Autodesk Fusion 360 part; units mm, degrees
(part 2 of 6)
  spline S17 degree 5 poles (13.6147, 25.8496) (13.6143, 25.8607) (13.6137, 25.8829) (13.6125, 25.9162) (13.6109, 25.9605) (13.6086, 26.0158) (13.6061, 26.0711) (13.6034, 26.1262) (13.6004, 26.1813) (13.5971, 26.2363) (13.5936, 26.2912) (13.5899, 26.346) (13.586, 26.4008) (13.5817, 26.4554) (13.5773, 26.51) (13.5726, 26.5644) (13.5676, 26.6188) (13.5624, 26.6731) (13.5569, 26.7273) (13.5512, 26.7813) (13.5453, 26.8353) (13.539, 26.8892) (13.5325, 26.943) (13.5258, 26.9966) (13.5188, 27.0502) (13.5115, 27.1037) (13.504, 27.157) (13.4962, 27.2102) (13.4882, 27.2634) (13.4798, 27.3164) (13.4712, 27.3693) (13.4623, 27.422) (13.4532, 27.4747) (13.4438, 27.5272) (13.4341, 27.5796) (13.4241, 27.6319) (13.4138, 27.684) (13.4032, 27.736) (13.3924, 27.7879) (13.3812, 27.8397) (13.3698, 27.8913) (13.3581, 27.9427) (13.346, 27.994) (13.3337, 28.0452) (13.321, 28.0962) (13.308, 28.147) (13.2947, 28.1977) (13.2811, 28.2483) (13.2672, 28.2986) (13.253, 28.3488) (13.2384, 28.3989) (13.2234, 28.4487) (13.2081, 28.4983) (13.1924, 28.5478) (13.1763, 28.597) (13.1599, 28.646) (13.1431, 28.6949) (13.126, 28.7436) (13.1086, 28.7921) (13.0908, 28.8403) (13.0724, 28.8883) (13.0536, 28.936) (13.0341, 28.9833) (13.014, 29.0303) (12.9935, 29.0769) (12.9725, 29.1234) (12.9513, 29.1696) (12.9298, 29.2157) (12.9079, 29.2615) (12.8852, 29.3069) (12.8613, 29.3515) (12.8409, 29.3863) (12.8246, 29.4119) (12.8134, 29.4287) (12.8076, 29.437) knots -1 -1 -1 -1 -1 -1 -0.98571429 -0.97142857 -0.95714286 -0.94285714 -0.92857143 -0.91428571 -0.9 -0.88571429 -0.87142857 -0.85714286 -0.84285714 -0.82857143 -0.81428571 -0.8 -0.78571429 -0.77142857 -0.75714286 -0.74285714 -0.72857143 -0.71428571 -0.7 -0.68571429 -0.67142857 -0.65714286 -0.64285714 -0.62857143 -0.61428571 -0.6 -0.58571429 -0.57142857 -0.55714286 -0.54285714 -0.52857143 -0.51428571 -0.5 -0.48571429 -0.47142857 -0.45714286 -0.44285714 -0.42857143 -0.41428571 -0.4 -0.38571429 -0.37142857 -0.35714286 -0.34285714 -0.32857143 -0.31428571 -0.3 -0.28571429 -0.27142857 -0.25714286 -0.24285714 -0.22857143 -0.21428571 -0.2 -0.18571429 -0.17142857 -0.15714286 -0.14285714 -0.12857143 -0.11428571 -0.1 -0.08571429 -0.07142857 -0.05714286 -0.04285714 -0.02857143 -0.01428571 0 0 0 0 0 0
  line L17 (12.8076, 29.437) -> (12.7927, 29.4587)
  arc A35 (13.0124, 30.8231) -> (12.7927, 29.4587) centre (13.6162, 30.026) ccw
  arc A36 (13.0124, 30.8231) -> (13.2238, 30.9853) centre (0, 48) ccw
  arc A37 (14.5985, 30.8444) -> (13.2238, 30.9853) centre (13.8374, 30.1957) ccw
  line L18 (14.5985, 30.8444) -> (14.6156, 30.8243)
  spline S18 degree 5 poles (14.6156, 30.8243) (14.6222, 30.8166) (14.6355, 30.8014) (14.656, 30.7791) (14.6843, 30.7503) (14.7212, 30.7157) (14.7592, 30.6821) (14.7977, 30.6491) (14.8367, 30.6164) (14.8759, 30.5839) (14.9153, 30.5516) (14.9551, 30.5197) (14.9953, 30.4881) (15.0359, 30.4571) (15.0771, 30.4265) (15.1187, 30.3964) (15.1607, 30.3667) (15.203, 30.3373) (15.2456, 30.3082) (15.2885, 30.2794) (15.3316, 30.2508) (15.375, 30.2225) (15.4187, 30.1946) (15.4626, 30.1669) (15.5069, 30.1396) (15.5514, 30.1125) (15.5963, 30.0858) (15.6413, 30.0593) (15.6866, 30.0331) (15.7321, 30.0071) (15.7779, 29.9814) (15.8239, 29.956) (15.8701, 29.9308) (15.9165, 29.9059) (15.9632, 29.8812) (16.0101, 29.8568) (16.0572, 29.8327) (16.1045, 29.8088) (16.152, 29.7851) (16.1997, 29.7617) (16.2476, 29.7385) (16.2957, 29.7156) (16.344, 29.6929) (16.3925, 29.6704) (16.4412, 29.6482) (16.49, 29.6262) (16.5391, 29.6044) (16.5883, 29.5829) (16.6377, 29.5616) (16.6873, 29.5405) (16.737, 29.5196) (16.787, 29.499) (16.8371, 29.4786) (16.8873, 29.4584) (16.9377, 29.4385) (16.9883, 29.4187) (17.0391, 29.3992) (17.09, 29.3799) (17.1411, 29.3608) (17.1923, 29.342) (17.2437, 29.3233) (17.2953, 29.3049) (17.3469, 29.2867) (17.3988, 29.2687) (17.4508, 29.2509) (17.5029, 29.2333) (17.5552, 29.216) (17.6076, 29.1988) (17.6602, 29.1819) (17.7129, 29.1652) (17.7658, 29.1486) (17.8081, 29.1356) (17.84, 29.1259) (17.8613, 29.1195) (17.8719, 29.1163) knots 0 0 0 0 0 0 0.01428571 0.02857143 0.04285714 0.05714286 0.07142857 0.08571429 0.1 0.11428571 0.12857143 0.14285714 0.15714286 0.17142857 0.18571429 0.2 0.21428571 0.22857143 0.24285714 0.25714286 0.27142857 0.28571429 0.3 0.31428571 0.32857143 0.34285714 0.35714286 0.37142857 0.38571429 0.4 0.41428571 0.42857143 0.44285714 0.45714286 0.47142857 0.48571429 0.5 0.51428571 0.52857143 0.54285714 0.55714286 0.57142857 0.58571429 0.6 0.61428571 0.62857143 0.64285714 0.65714286 0.67142857 0.68571429 0.7 0.71428571 0.72857143 0.74285714 0.75714286 0.77142857 0.78571429 0.8 0.81428571 0.82857143 0.84285714 0.85714286 0.87142857 0.88571429 0.9 0.91428571 0.92857143 0.94285714 0.95714286 0.97142857 0.98571429 1 1 1 1 1 1
  arc A38 (17.8719, 29.1163) -> (18.8837, 30.1281) centre (0, 48) ccw
  spline S19 degree 5 poles (18.8837, 30.1281) (18.8805, 30.1387) (18.8741, 30.16) (18.8644, 30.1919) (18.8514, 30.2342) (18.8348, 30.2871) (18.8181, 30.3398) (18.8012, 30.3924) (18.784, 30.4448) (18.7667, 30.4971) (18.7491, 30.5492) (18.7313, 30.6012) (18.7133, 30.6531) (18.6951, 30.7047) (18.6767, 30.7563) (18.658, 30.8077) (18.6392, 30.8589) (18.6201, 30.91) (18.6008, 30.9609) (18.5813, 31.0117) (18.5615, 31.0623) (18.5416, 31.1127) (18.5214, 31.1629) (18.501, 31.213) (18.4804, 31.263) (18.4595, 31.3127) (18.4384, 31.3623) (18.4171, 31.4117) (18.3956, 31.4609) (18.3738, 31.51) (18.3518, 31.5588) (18.3296, 31.6075) (18.3071, 31.656) (18.2844, 31.7043) (18.2615, 31.7524) (18.2383, 31.8003) (18.2149, 31.848) (18.1912, 31.8955) (18.1673, 31.9428) (18.1432, 31.9899) (18.1188, 32.0368) (18.0941, 32.0835) (18.0692, 32.1299) (18.044, 32.1761) (18.0186, 32.2221) (17.9929, 32.2679) (17.9669, 32.3134) (17.9407, 32.3587) (17.9142, 32.4037) (17.8875, 32.4486) (17.8604, 32.4931) (17.8331, 32.5374) (17.8054, 32.5813) (17.7775, 32.625) (17.7492, 32.6684) (17.7206, 32.7115) (17.6918, 32.7544) (17.6627, 32.797) (17.6333, 32.8393) (17.6036, 32.8813) (17.5735, 32.9229) (17.5429, 32.9641) (17.5119, 33.0047) (17.4803, 33.0449) (17.4484, 33.0847) (17.4161, 33.1241) (17.3836, 33.1633) (17.3509, 33.2023) (17.3179, 33.2408) (17.2843, 33.2788) (17.2497, 33.3157) (17.2209, 33.344) (17.1986, 33.3645) (17.1834, 33.3778) (17.1757, 33.3844) knots -1 -1 -1 -1 -1 -1 -0.98571429 -0.97142857 -0.95714286 -0.94285714 -0.92857143 -0.91428571 -0.9 -0.88571429 -0.87142857 -0.85714286 -0.84285714 -0.82857143 -0.81428571 -0.8 -0.78571429 -0.77142857 -0.75714286 -0.74285714 -0.72857143 -0.71428571 -0.7 -0.68571429 -0.67142857 -0.65714286 -0.64285714 -0.62857143 -0.61428571 -0.6 -0.58571429 -0.57142857 -0.55714286 -0.54285714 -0.52857143 -0.51428571 -0.5 -0.48571429 -0.47142857 -0.45714286 -0.44285714 -0.42857143 -0.41428571 -0.4 -0.38571429 -0.37142857 -0.35714286 -0.34285714 -0.32857143 -0.31428571 -0.3 -0.28571429 -0.27142857 -0.25714286 -0.24285714 -0.22857143 -0.21428571 -0.2 -0.18571429 -0.17142857 -0.15714286 -0.14285714 -0.12857143 -0.11428571 -0.1 -0.08571429 -0.07142857 -0.05714286 -0.04285714 -0.02857143 -0.01428571 0 0 0 0 0 0
  line L19 (17.1757, 33.3844) -> (17.1556, 33.4015)
  arc A39 (17.0147, 34.7762) -> (17.1556, 33.4015) centre (17.8043, 34.1626) ccw
  arc A40 (17.0147, 34.7762) -> (17.1769, 34.9876) centre (0, 48) ccw
  arc A41 (18.5413, 35.2073) -> (17.1769, 34.9876) centre (17.974, 34.3838) ccw
  line L20 (18.5413, 35.2073) -> (18.563, 35.1924)
  spline S20 degree 5 poles (18.563, 35.1924) (18.5713, 35.1866) (18.5881, 35.1754) (18.6137, 35.1591) (18.6485, 35.1387) (18.6931, 35.1148) (18.7385, 35.0921) (18.7843, 35.0702) (18.8304, 35.0487) (18.8766, 35.0275) (18.9231, 35.0065) (18.9697, 34.986) (19.0167, 34.9659) (19.064, 34.9464) (19.1117, 34.9276) (19.1597, 34.9092) (19.2079, 34.8914) (19.2564, 34.874) (19.3051, 34.8569) (19.354, 34.8401) (19.403, 34.8237) (19.4522, 34.8076) (19.5017, 34.7919) (19.5513, 34.7766) (19.6011, 34.7616) (19.6512, 34.747) (19.7014, 34.7328) (19.7517, 34.7189) (19.8023, 34.7053) (19.853, 34.692) (19.9038, 34.679) (19.9548, 34.6663) (20.006, 34.654) (20.0573, 34.6419) (20.1087, 34.6302) (20.1603, 34.6188) (20.2121, 34.6076) (20.264, 34.5968) (20.316, 34.5862) (20.3681, 34.5759) (20.4204, 34.5659) (20.4728, 34.5562) (20.5253, 34.5468) (20.578, 34.5377) (20.6307, 34.5288) (20.6836, 34.5202) (20.7366, 34.5118) (20.7898, 34.5038) (20.843, 34.496) (20.8963, 34.4885) (20.9498, 34.4812) (21.0034, 34.4742) (21.057, 34.4675) (21.1108, 34.461) (21.1647, 34.4547) (21.2187, 34.4488) (21.2727, 34.4431) (21.3269, 34.4376) (21.3812, 34.4324) (21.4356, 34.4274) (21.49, 34.4227) (21.5446, 34.4183) (21.5992, 34.414) (21.654, 34.4101) (21.7088, 34.4064) (21.7637, 34.4029) (21.8187, 34.3996) (21.8738, 34.3966) (21.9289, 34.3939) (21.9842, 34.3914) (22.0395, 34.3891) (22.0838, 34.3875) (22.1171, 34.3863) (22.1393, 34.3857) (22.1504, 34.3853) knots 0 0 0 0 0 0 0.01428571 0.02857143 0.04285714 0.05714286 0.07142857 0.08571429 0.1 0.11428571 0.12857143 0.14285714 0.15714286 0.17142857 0.18571429 0.2 0.21428571 0.22857143 0.24285714 0.25714286 0.27142857 0.28571429 0.3 0.31428571 0.32857143 0.34285714 0.35714286 0.37142857 0.38571429 0.4 0.41428571 0.42857143 0.44285714 0.45714286 0.47142857 0.48571429 0.5 0.51428571 0.52857143 0.54285714 0.55714286 0.57142857 0.58571429 0.6 0.61428571 0.62857143 0.64285714 0.65714286 0.67142857 0.68571429 0.7 0.71428571 0.72857143 0.74285714 0.75714286 0.77142857 0.78571429 0.8 0.81428571 0.82857143 0.84285714 0.85714286 0.87142857 0.88571429 0.9 0.91428571 0.92857143 0.94285714 0.95714286 0.97142857 0.98571429 1 1 1 1 1 1
  arc A42 (22.1504, 34.3853) -> (22.8659, 35.6245) centre (0, 48) ccw
  spline S21 degree 5 poles (22.8659, 35.6245) (22.86, 35.634) (22.8483, 35.6529) (22.8307, 35.6811) (22.8071, 35.7187) (22.7775, 35.7655) (22.7477, 35.812) (22.7177, 35.8584) (22.6876, 35.9046) (22.6573, 35.9507) (22.6268, 35.9965) (22.5962, 36.0421) (22.5654, 36.0875) (22.5344, 36.1327) (22.5033, 36.1777) (22.472, 36.2225) (22.4405, 36.2671) (22.4088, 36.3115) (22.377, 36.3557) (22.345, 36.3997) (22.3129, 36.4435) (22.2805, 36.487) (22.248, 36.5303) (22.2154, 36.5735) (22.1825, 36.6163) (22.1495, 36.659) (22.1163, 36.7014) (22.0829, 36.7436) (22.0494, 36.7856) (22.0157, 36.8274) (21.9818, 36.8689) (21.9477, 36.9101) (21.9135, 36.9512) (21.879, 36.9919) (21.8444, 37.0325) (21.8096, 37.0727) (21.7747, 37.1127) (21.7395, 37.1525) (21.7042, 37.192) (21.6687, 37.2313) (21.633, 37.2702) (21.5971, 37.3089) (21.561, 37.3473) (21.5247, 37.3854) (21.4882, 37.4233) (21.4516, 37.4608) (21.4147, 37.4981) (21.3777, 37.5351) (21.3404, 37.5717) (21.303, 37.6081) (21.2653, 37.6441) (21.2275, 37.6798) (21.1894, 37.7151) (21.1511, 37.7501) (21.1125, 37.7847) (21.0738, 37.8189) (21.0348, 37.8529) (20.9957, 37.8865) (20.9563, 37.9197) (20.9168, 37.9526) (20.8769, 37.985) (20.8367, 38.0168) (20.7962, 38.0481) (20.7554, 38.0787) (20.7142, 38.1089) (20.6728, 38.1386) (20.6313, 38.1681) (20.5897, 38.1972) (20.5478, 38.2259) (20.5055, 38.2539) (20.4625, 38.2806) (20.4274, 38.3005) (20.4005, 38.3145) (20.3824, 38.3235) (20.3732, 38.3278) knots -1 -1 -1 -1 -1 -1 -0.98571429 -0.97142857 -0.95714286 -0.94285714 -0.92857143 -0.91428571 -0.9 -0.88571429 -0.87142857 -0.85714286 -0.84285714 -0.82857143 -0.81428571 -0.8 -0.78571429 -0.77142857 -0.75714286 -0.74285714 -0.72857143 -0.71428571 -0.7 -0.68571429 -0.67142857 -0.65714286 -0.64285714 -0.62857143 -0.61428571 -0.6 -0.58571429 -0.57142857 -0.55714286 -0.54285714 -0.52857143 -0.51428571 -0.5 -0.48571429 -0.47142857 -0.45714286 -0.44285714 -0.42857143 -0.41428571 -0.4 -0.38571429 -0.37142857 -0.35714286 -0.34285714 -0.32857143 -0.31428571 -0.3 -0.28571429 -0.27142857 -0.25714286 -0.24285714 -0.22857143 -0.21428571 -0.2 -0.18571429 -0.17142857 -0.15714286 -0.14285714 -0.12857143 -0.11428571 -0.1 -0.08571429 -0.07142857 -0.05714286 -0.04285714 -0.02857143 -0.01428571 0 0 0 0 0 0
  line L21 (20.3732, 38.3278) -> (20.3494, 38.3391)
  arc A43 (19.8575, 39.6305) -> (20.3494, 38.3391) centre (20.779, 39.2422) ccw
  arc A44 (19.8575, 39.6305) -> (19.9595, 39.8767) centre (0, 48) ccw
  arc A45 (21.2205, 40.4421) -> (19.9595, 39.8767) centre (20.8857, 39.4998) ccw
  line L22 (21.2205, 40.4421) -> (21.2453, 40.4332)
  spline S22 degree 5 poles (21.2453, 40.4332) (21.2549, 40.4298) (21.274, 40.4233) (21.3029, 40.4142) (21.3419, 40.4035) (21.3911, 40.392) (21.4408, 40.3818) (21.4907, 40.3725) (21.5408, 40.3637) (21.591, 40.3551) (21.6412, 40.3469) (21.6916, 40.3391) (21.7422, 40.3319) (21.7929, 40.3254) (21.8439, 40.3195) (21.895, 40.3142) (21.9462, 40.3094) (21.9975, 40.3052) (22.049, 40.3012) (22.1005, 40.2977) (22.1521, 40.2945) (22.2039, 40.2917) (22.2557, 40.2894) (22.3076, 40.2874) (22.3596, 40.2859) (22.4117, 40.2847) (22.4639, 40.2839) (22.5161, 40.2835) (22.5685, 40.2835) (22.6209, 40.2838) (22.6733, 40.2844) (22.7259, 40.2854) (22.7785, 40.2867) (22.8312, 40.2883) (22.8839, 40.2903) (22.9367, 40.2926) (22.9896, 40.2952) (23.0425, 40.2982) (23.0955, 40.3014) (23.1485, 40.305) (23.2016, 40.3089) (23.2547, 40.3131) (23.3079, 40.3176) (23.3611, 40.3223) (23.4144, 40.3274) (23.4677, 40.3328) (23.521, 40.3385) (23.5744, 40.3444) (23.6279, 40.3507) (23.6814, 40.3572) (23.7349, 40.364) (23.7884, 40.3711) (23.842, 40.3785) (23.8956, 40.3862) (23.9493, 40.3941) (24.003, 40.4023) (24.0567, 40.4108) (24.1104, 40.4195) (24.1642, 40.4286) (24.218, 40.4378) (24.2718, 40.4474) (24.3257, 40.4572) (24.3796, 40.4673) (24.4335, 40.4776) (24.4874, 40.4882) (24.5413, 40.499) (24.5953, 40.5101) (24.6492, 40.5215) (24.7032, 40.5331) (24.7573, 40.545) (24.8113, 40.5571) (24.8545, 40.567) (24.8869, 40.5745) (24.9086, 40.5796) (24.9194, 40.5822) knots 0 0 0 0 0 0 0.01428571 0.02857143 0.04285714 0.05714286 0.07142857 0.08571429 0.1 0.11428571 0.12857143 0.14285714 0.15714286 0.17142857 0.18571429 0.2 0.21428571 0.22857143 0.24285714 0.25714286 0.27142857 0.28571429 0.3 0.31428571 0.32857143 0.34285714 0.35714286 0.37142857 0.38571429 0.4 0.41428571 0.42857143 0.44285714 0.45714286 0.47142857 0.48571429 0.5 0.51428571 0.52857143 0.54285714 0.55714286 0.57142857 0.58571429 0.6 0.61428571 0.62857143 0.64285714 0.65714286 0.67142857 0.68571429 0.7 0.71428571 0.72857143 0.74285714 0.75714286 0.77142857 0.78571429 0.8 0.81428571 0.82857143 0.84285714 0.85714286 0.87142857 0.88571429 0.9 0.91428571 0.92857143 0.94285714 0.95714286 0.97142857 0.98571429 1 1 1 1 1 1
  arc A46 (24.9194, 40.5822) -> (25.2897, 41.9643) centre (0, 48) ccw
  spline S23 degree 5 poles (25.2897, 41.9643) (25.2816, 41.9719) (25.2655, 41.9872) (25.2411, 42.0099) (25.2086, 42.0401) (25.1679, 42.0776) (25.1271, 42.1149) (25.0861, 42.1519) (25.0451, 42.1888) (25.0039, 42.2254) (24.9626, 42.2617) (24.9212, 42.2979) (24.8797, 42.3338) (24.8381, 42.3694) (24.7963, 42.4048) (24.7545, 42.44) (24.7125, 42.475) (24.6705, 42.5097) (24.6283, 42.5441) (24.586, 42.5783) (24.5436, 42.6122) (24.5011, 42.6459) (24.4585, 42.6794) (24.4158, 42.7126) (24.373, 42.7455) (24.33, 42.7782) (24.287, 42.8105) (24.2438, 42.8427) (24.2006, 42.8745) (24.1572, 42.9061) (24.1137, 42.9375) (24.0701, 42.9685) (24.0264, 42.9993) (23.9826, 43.0297) (23.9387, 43.0599) (23.8947, 43.0898) (23.8505, 43.1194) (23.8063, 43.1487) (23.7619, 43.1777) (23.7175, 43.2065) (23.6729, 43.2349) (23.6282, 43.2629) (23.5834, 43.2907) (23.5385, 43.3181) (23.4935, 43.3452) (23.4484, 43.372) (23.4031, 43.3985) (23.3578, 43.4246) (23.3123, 43.4504) (23.2667, 43.4758) (23.221, 43.5008) (23.1752, 43.5255) (23.1293, 43.5498) (23.0832, 43.5736) (23.037, 43.5971) (22.9908, 43.6201) (22.9444, 43.6428) (22.8979, 43.6652) (22.8512, 43.6871) (22.8045, 43.7086) (22.7576, 43.7296) (22.7106, 43.75) (22.6633, 43.7696) (22.6159, 43.7887) (22.5684, 43.8071) (22.5207, 43.8252) (22.473, 43.8429) (22.4252, 43.8602) (22.3773, 43.8771) (22.3292, 43.8932) (22.2808, 43.9078) (22.2417, 43.918) (22.2122, 43.9246) (22.1923, 43.9285) (22.1824, 43.9304) knots -1 -1 -1 -1 -1 -1 -0.98571429 -0.97142857 -0.95714286 -0.94285714 -0.92857143 -0.91428571 -0.9 -0.88571429 -0.87142857 -0.85714286 -0.84285714 -0.82857143 -0.81428571 -0.8 -0.78571429 -0.77142857 -0.75714286 -0.74285714 -0.72857143 -0.71428571 -0.7 -0.68571429 -0.67142857 -0.65714286 -0.64285714 -0.62857143 -0.61428571 -0.6 -0.58571429 -0.57142857 -0.55714286 -0.54285714 -0.52857143 -0.51428571 -0.5 -0.48571429 -0.47142857 -0.45714286 -0.44285714 -0.42857143 -0.41428571 -0.4 -0.38571429 -0.37142857 -0.35714286 -0.34285714 -0.32857143 -0.31428571 -0.3 -0.28571429 -0.27142857 -0.25714286 -0.24285714 -0.22857143 -0.21428571 -0.2 -0.18571429 -0.17142857 -0.15714286 -0.14285714 -0.12857143 -0.11428571 -0.1 -0.08571429 -0.07142857 -0.05714286 -0.04285714 -0.02857143 -0.01428571 0 0 0 0 0 0
  line L23 (22.1824, 43.9304) -> (22.1564, 43.9351)
  arc A47 (21.347, 45.0552) -> (22.1564, 43.9351) centre (22.3377, 44.9186) ccw
  arc A48 (21.347, 45.0552) -> (21.3818, 45.3194) centre (0, 48) ccw
  arc A49 (22.4535, 46.1918) -> (21.3818, 45.3194) centre (22.3741, 45.195) ccw
  line L24 (22.4535, 46.1918) -> (22.4799, 46.1898)
  spline S24 degree 5 poles (22.4799, 46.1898) (22.4899, 46.1889) (22.5101, 46.1876) (22.5404, 46.1863) (22.5808, 46.186) (22.6313, 46.1877) (22.6819, 46.1907) (22.7326, 46.1946) (22.7832, 46.199) (22.8339, 46.2038) (22.8846, 46.2089) (22.9353, 46.2144) (22.986, 46.2205) (23.0367, 46.2273) (23.0874, 46.2348) (23.1381, 46.2429) (23.1889, 46.2516) (23.2396, 46.2607) (23.2903, 46.2703) (23.341, 46.2802) (23.3916, 46.2905) (23.4423, 46.3012) (23.493, 46.3123) (23.5436, 46.3238) (23.5943, 46.3358) (23.6449, 46.3482) (23.6955, 46.3609) (23.7461, 46.3741) (23.7966, 46.3876) (23.8472, 46.4014) (23.8977, 46.4156) (23.9482, 46.4301) (23.9987, 46.445) (24.0491, 46.4602) (24.0996, 46.4758) (24.15, 46.4917) (24.2004, 46.5079) (24.2507, 46.5244) (24.301, 46.5413) (24.3513, 46.5585) (24.4016, 46.576) (24.4518, 46.5938) (24.502, 46.6119) (24.5522, 46.6303) (24.6024, 46.649) (24.6525, 46.6679) (24.7025, 46.6872) (24.7526, 46.7068) (24.8026, 46.7267) (24.8525, 46.7468) (24.9025, 46.7673) (24.9523, 46.788) (25.0022, 46.809) (25.052, 46.8303) (25.1018, 46.8518) (25.1515, 46.8736) (25.2012, 46.8957) (25.2509, 46.9181) (25.3005, 46.9407) (25.35, 46.9636) (25.3995, 46.9867) (25.449, 47.0102) (25.4985, 47.0338) (25.5478, 47.0578) (25.5972, 47.0819) (25.6465, 47.1064) (25.6957, 47.1311) (25.7449, 47.156) (25.7941, 47.1812) (25.8432, 47.2067) (25.8922, 47.2324) (25.9314, 47.2531) (25.9608, 47.2688) (25.9804, 47.2793) (25.9902, 47.2845) knots 0 0 0 0 0 0 0.01428571 0.02857143 0.04285714 0.05714286 0.07142857 0.08571429 0.1 0.11428571 0.12857143 0.14285714 0.15714286 0.17142857 0.18571429 0.2 0.21428571 0.22857143 0.24285714 0.25714286 0.27142857 0.28571429 0.3 0.31428571 0.32857143 0.34285714 0.35714286 0.37142857 0.38571429 0.4 0.41428571 0.42857143 0.44285714 0.45714286 0.47142857 0.48571429 0.5 0.51428571 0.52857143 0.54285714 0.55714286 0.57142857 0.58571429 0.6 0.61428571 0.62857143 0.64285714 0.65714286 0.67142857 0.68571429 0.7 0.71428571 0.72857143 0.74285714 0.75714286 0.77142857 0.78571429 0.8 0.81428571 0.82857143 0.84285714 0.85714286 0.87142857 0.88571429 0.9 0.91428571 0.92857143 0.94285714 0.95714286 0.97142857 0.98571429 1 1 1 1 1 1
  arc A50 (25.9902, 47.2845) -> (25.9902, 48.7155) centre (0, 48) ccw
  spline S25 degree 5 poles (25.9902, 48.7155) (25.9804, 48.7207) (25.9608, 48.7312) (25.9314, 48.7469) (25.8922, 48.7676) (25.8432, 48.7933) (25.7941, 48.8188) (25.7449, 48.844) (25.6957, 48.8689) (25.6465, 48.8936) (25.5972, 48.9181) (25.5478, 48.9422) (25.4985, 48.9662) (25.449, 48.9898) (25.3995, 49.0133) (25.35, 49.0364) (25.3005, 49.0593) (25.2509, 49.0819) (25.2012, 49.1043) (25.1515, 49.1264) (25.1018, 49.1482) (25.052, 49.1697) (25.0022, 49.191) (24.9523, 49.212) (24.9025, 49.2327) (24.8525, 49.2532) (24.8026, 49.2733) (24.7526, 49.2932) (24.7025, 49.3128) (24.6525, 49.3321) (24.6024, 49.351) (24.5522, 49.3697) (24.502, 49.3881) (24.4518, 49.4062) (24.4016, 49.424) (24.3513, 49.4415) (24.301, 49.4587) (24.2507, 49.4756) (24.2004, 49.4921) (24.15, 49.5083) (24.0996, 49.5242) (24.0491, 49.5398) (23.9987, 49.555) (23.9482, 49.5699) (23.8977, 49.5844) (23.8472, 49.5986) (23.7966, 49.6124) (23.7461, 49.6259) (23.6955, 49.6391) (23.6449, 49.6518) (23.5943, 49.6642) (23.5436, 49.6762) (23.493, 49.6877) (23.4423, 49.6988) (23.3916, 49.7095) (23.341, 49.7198) (23.2903, 49.7297) (23.2396, 49.7393) (23.1889, 49.7484) (23.1381, 49.7571) (23.0874, 49.7652) (23.0367, 49.7727) (22.986, 49.7795) (22.9353, 49.7856) (22.8846, 49.7911) (22.8339, 49.7962) (22.7832, 49.801) (22.7326, 49.8054) (22.6819, 49.8093) (22.6313, 49.8123) (22.5808, 49.814) (22.5404, 49.8137) (22.5101, 49.8124) (22.4899, 49.8111) (22.4799, 49.8102) knots -1 -1 -1 -1 -1 -1 -0.98571429 -0.97142857 -0.95714286 -0.94285714 -0.92857143 -0.91428571 -0.9 -0.88571429 -0.87142857 -0.85714286 -0.84285714 -0.82857143 -0.81428571 -0.8 -0.78571429 -0.77142857 -0.75714286 -0.74285714 -0.72857143 -0.71428571 -0.7 -0.68571429 -0.67142857 -0.65714286 -0.64285714 -0.62857143 -0.61428571 -0.6 -0.58571429 -0.57142857 -0.55714286 -0.54285714 -0.52857143 -0.51428571 -0.5 -0.48571429 -0.47142857 -0.45714286 -0.44285714 -0.42857143 -0.41428571 -0.4 -0.38571429 -0.37142857 -0.35714286 -0.34285714 -0.32857143 -0.31428571 -0.3 -0.28571429 -0.27142857 -0.25714286 -0.24285714 -0.22857143 -0.21428571 -0.2 -0.18571429 -0.17142857 -0.15714286 -0.14285714 -0.12857143 -0.11428571 -0.1 -0.08571429 -0.07142857 -0.05714286 -0.04285714 -0.02857143 -0.01428571 0 0 0 0 0 0
  line L25 (22.4799, 49.8102) -> (22.4535, 49.8082)
  arc A51 (21.3818, 50.6806) -> (22.4535, 49.8082) centre (22.3741, 50.805) ccw
  arc A52 (21.3818, 50.6806) -> (21.347, 50.9448) centre (0, 48) ccw
  arc A53 (22.1564, 52.0649) -> (21.347, 50.9448) centre (22.3377, 51.0814) ccw
  line L26 (22.1564, 52.0649) -> (22.1824, 52.0696)
  spline S26 degree 5 poles (22.1824, 52.0696) (22.1923, 52.0715) (22.2122, 52.0754) (22.2417, 52.082) (22.2808, 52.0922) (22.3292, 52.1068) (22.3773, 52.1229) (22.4252, 52.1398) (22.473, 52.1571) (22.5207, 52.1748) (22.5684, 52.1929) (22.6159, 52.2113) (22.6633, 52.2304) (22.7106, 52.25) (22.7576, 52.2704) (22.8045, 52.2914) (22.8512, 52.3129) (22.8979, 52.3348) (22.9444, 52.3572) (22.9908, 52.3799) (23.037, 52.4029) (23.0832, 52.4264) (23.1293, 52.4502) (23.1752, 52.4745) (23.221, 52.4992) (23.2667, 52.5242) (23.3123, 52.5496) (23.3578, 52.5754) (23.4031, 52.6015) (23.4484, 52.628) (23.4935, 52.6548) (23.5385, 52.6819) (23.5834, 52.7093) (23.6282, 52.7371) (23.6729, 52.7651) (23.7175, 52.7935) (23.7619, 52.8223) (23.8063, 52.8513) (23.8505, 52.8806) (23.8947, 52.9102) (23.9387, 52.9401) (23.9826, 52.9703) (24.0264, 53.0007) (24.0701, 53.0315) (24.1137, 53.0625) (24.1572, 53.0939) (24.2006, 53.1255) (24.2438, 53.1573) (24.287, 53.1895) (24.33, 53.2218) (24.373, 53.2545) (24.4158, 53.2874) (24.4585, 53.3206) (24.5011, 53.3541) (24.5436, 53.3878) (24.586, 53.4217) (24.6283, 53.4559) (24.6705, 53.4903) (24.7125, 53.525) (24.7545, 53.56) (24.7963, 53.5952) (24.8381, 53.6306) (24.8797, 53.6662) (24.9212, 53.7021) (24.9626, 53.7383) (25.0039, 53.7746) (25.0451, 53.8112) (25.0861, 53.8481) (25.1271, 53.8851) (25.1679, 53.9224) (25.2086, 53.9599) (25.2411, 53.9901) (25.2655, 54.0128) (25.2816, 54.0281) (25.2897, 54.0357) knots 0 0 0 0 0 0 0.01428571 0.02857143 0.04285714 0.05714286 0.07142857 0.08571429 0.1 0.11428571 0.12857143 0.14285714 0.15714286 0.17142857 0.18571429 0.2 0.21428571 0.22857143 0.24285714 0.25714286 0.27142857 0.28571429 0.3 0.31428571 0.32857143 0.34285714 0.35714286 0.37142857 0.38571429 0.4 0.41428571 0.42857143 0.44285714 0.45714286 0.47142857 0.48571429 0.5 0.51428571 0.52857143 0.54285714 0.55714286 0.57142857 0.58571429 0.6 0.61428571 0.62857143 0.64285714 0.65714286 0.67142857 0.68571429 0.7 0.71428571 0.72857143 0.74285714 0.75714286 0.77142857 0.78571429 0.8 0.81428571 0.82857143 0.84285714 0.85714286 0.87142857 0.88571429 0.9 0.91428571 0.92857143 0.94285714 0.95714286 0.97142857 0.98571429 1 1 1 1 1 1
  arc A54 (25.2897, 54.0357) -> (24.9194, 55.4178) centre (0, 48) ccw
  spline S27 degree 5 poles (24.9194, 55.4178) (24.9086, 55.4204) (24.8869, 55.4255) (24.8545, 55.433) (24.8113, 55.4429) (24.7573, 55.455) (24.7032, 55.4669) (24.6492, 55.4785) (24.5953, 55.4899) (24.5413, 55.501) (24.4874, 55.5118) (24.4335, 55.5224) (24.3796, 55.5327) (24.3257, 55.5428) (24.2718, 55.5526) (24.218, 55.5622) (24.1642, 55.5714) (24.1104, 55.5805) (24.0567, 55.5892) (24.003, 55.5977) (23.9493, 55.6059) (23.8956, 55.6138) (23.842, 55.6215) (23.7884, 55.6289) (23.7349, 55.636) (23.6814, 55.6428) (23.6279, 55.6493) (23.5744, 55.6556) (23.521, 55.6615) (23.4677, 55.6672) (23.4144, 55.6726) (23.3611, 55.6777) (23.3079, 55.6824) (23.2547, 55.6869) (23.2016, 55.6911) (23.1485, 55.695) (23.0955, 55.6986) (23.0425, 55.7018) (22.9896, 55.7048) (22.9367, 55.7074) (22.8839, 55.7097) (22.8312, 55.7117) (22.7785, 55.7133) (22.7259, 55.7146) (22.6733, 55.7156) (22.6209, 55.7162) (22.5685, 55.7165) (22.5161, 55.7165) (22.4639, 55.7161) (22.4117, 55.7153) (22.3596, 55.7141) (22.3076, 55.7126) (22.2557, 55.7106) (22.2039, 55.7083) (22.1521, 55.7055) (22.1005, 55.7023) (22.049, 55.6988) (21.9975, 55.6948) (21.9462, 55.6906) (21.895, 55.6858) (21.8439, 55.6805) (21.7929, 55.6746) (21.7422, 55.6681) (21.6916, 55.6609) (21.6412, 55.6531) (21.591, 55.6449) (21.5408, 55.6363) (21.4907, 55.6275) (21.4408, 55.6182) (21.3911, 55.608) (21.3419, 55.5965) (21.3029, 55.5858) (21.274, 55.5767) (21.2549, 55.5702) (21.2453, 55.5668) knots -1 -1 -1 -1 -1 -1 -0.98571429 -0.97142857 -0.95714286 -0.94285714 -0.92857143 -0.91428571 -0.9 -0.88571429 -0.87142857 -0.85714286 -0.84285714 -0.82857143 -0.81428571 -0.8 -0.78571429 -0.77142857 -0.75714286 -0.74285714 -0.72857143 -0.71428571 -0.7 -0.68571429 -0.67142857 -0.65714286 -0.64285714 -0.62857143 -0.61428571 -0.6 -0.58571429 -0.57142857 -0.55714286 -0.54285714 -0.52857143 -0.51428571 -0.5 -0.48571429 -0.47142857 -0.45714286 -0.44285714 -0.42857143 -0.41428571 -0.4 -0.38571429 -0.37142857 -0.35714286 -0.34285714 -0.32857143 -0.31428571 -0.3 -0.28571429 -0.27142857 -0.25714286 -0.24285714 -0.22857143 -0.21428571 -0.2 -0.18571429 -0.17142857 -0.15714286 -0.14285714 -0.12857143 -0.11428571 -0.1 -0.08571429 -0.07142857 -0.05714286 -0.04285714 -0.02857143 -0.01428571 0 0 0 0 0 0
  line L27 (21.2453, 55.5668) -> (21.2205, 55.5579)
  arc A55 (19.9595, 56.1233) -> (21.2205, 55.5579) centre (20.8857, 56.5002) ccw
  arc A56 (19.9595, 56.1233) -> (19.8575, 56.3695) centre (0, 48) ccw
  arc A57 (20.3494, 57.6609) -> (19.8575, 56.3695) centre (20.779, 56.7578) ccw
  line L28 (20.3494, 57.6609) -> (20.3732, 57.6722)
  spline S28 degree 5 poles (20.3732, 57.6722) (20.3824, 57.6765) (20.4005, 57.6855) (20.4274, 57.6995) (20.4625, 57.7194) (20.5055, 57.7461) (20.5478, 57.7741) (20.5897, 57.8028) (20.6313, 57.8319) (20.6728, 57.8614) (20.7142, 57.8911) (20.7554, 57.9213) (20.7962, 57.9519) (20.8367, 57.9832) (20.8769, 58.015) (20.9168, 58.0474) (20.9563, 58.0803) (20.9957, 58.1135) (21.0348, 58.1471) (21.0738, 58.1811) (21.1125, 58.2153) (21.1511, 58.2499) (21.1894, 58.2849) (21.2275, 58.3202) (21.2653, 58.3559) (21.303, 58.3919) (21.3404, 58.4283) (21.3777, 58.4649) (21.4147, 58.5019) (21.4516, 58.5392) (21.4882, 58.5767) (21.5247, 58.6146) (21.561, 58.6527) (21.5971, 58.6911) (21.633, 58.7298) (21.6687, 58.7687) (21.7042, 58.808) (21.7395, 58.8475) (21.7747, 58.8873) (21.8096, 58.9273) (21.8444, 58.9675) (21.879, 59.0081) (21.9135, 59.0488) (21.9477, 59.0899) (21.9818, 59.1311) (22.0157, 59.1726) (22.0494, 59.2144) (22.0829, 59.2564) (22.1163, 59.2986) (22.1495, 59.341) (22.1825, 59.3837) (22.2154, 59.4265) (22.248, 59.4697) (22.2805, 59.513) (22.3129, 59.5565) (22.345, 59.6003) (22.377, 59.6443) (22.4088, 59.6885) (22.4405, 59.7329) (22.472, 59.7775) (22.5033, 59.8223) (22.5344, 59.8673) (22.5654, 59.9125) (22.5962, 59.9579) (22.6268, 60.0035) (22.6573, 60.0493) (22.6876, 60.0954) (22.7177, 60.1416) (22.7477, 60.188) (22.7775, 60.2345) (22.8071, 60.2813) (22.8307, 60.3189) (22.8483, 60.3471) (22.86, 60.366) (22.8659, 60.3755) knots 0 0 0 0 0 0 0.01428571 0.02857143 0.04285714 0.05714286 0.07142857 0.08571429 0.1 0.11428571 0.12857143 0.14285714 0.15714286 0.17142857 0.18571429 0.2 0.21428571 0.22857143 0.24285714 0.25714286 0.27142857 0.28571429 0.3 0.31428571 0.32857143 0.34285714 0.35714286 0.37142857 0.38571429 0.4 0.41428571 0.42857143 0.44285714 0.45714286 0.47142857 0.48571429 0.5 0.51428571 0.52857143 0.54285714 0.55714286 0.57142857 0.58571429 0.6 0.61428571 0.62857143 0.64285714 0.65714286 0.67142857 0.68571429 0.7 0.71428571 0.72857143 0.74285714 0.75714286 0.77142857 0.78571429 0.8 0.81428571 0.82857143 0.84285714 0.85714286 0.87142857 0.88571429 0.9 0.91428571 0.92857143 0.94285714 0.95714286 0.97142857 0.98571429 1 1 1 1 1 1
  arc A58 (22.8659, 60.3755) -> (22.1504, 61.6147) centre (0, 48) ccw
  spline S29 degree 5 poles (22.1504, 61.6147) (22.1393, 61.6143) (22.1171, 61.6137) (22.0838, 61.6125) (22.0395, 61.6109) (21.9842, 61.6086) (21.9289, 61.6061) (21.8738, 61.6034) (21.8187, 61.6004) (21.7637, 61.5971) (21.7088, 61.5936) (21.654, 61.5899) (21.5992, 61.586) (21.5446, 61.5817) (21.49, 61.5773) (21.4356, 61.5726) (21.3812, 61.5676) (21.3269, 61.5624) (21.2727, 61.5569) (21.2187, 61.5512) (21.1647, 61.5453) (21.1108, 61.539) (21.057, 61.5325) (21.0034, 61.5258) (20.9498, 61.5188) (20.8963, 61.5115) (20.843, 61.504) (20.7898, 61.4962) (20.7366, 61.4882) (20.6836, 61.4798) (20.6307, 61.4712) (20.578, 61.4623) (20.5253, 61.4532) (20.4728, 61.4438) (20.4204, 61.4341) (20.3681, 61.4241) (20.316, 61.4138) (20.264, 61.4032) (20.2121, 61.3924) (20.1603, 61.3812) (20.1087, 61.3698) (20.0573, 61.3581) (20.006, 61.346) (19.9548, 61.3337) (19.9038, 61.321) (19.853, 61.308) (19.8023, 61.2947) (19.7517, 61.2811) (19.7014, 61.2672) (19.6512, 61.253) (19.6011, 61.2384) (19.5513, 61.2234) (19.5017, 61.2081) (19.4522, 61.1924) (19.403, 61.1763) (19.354, 61.1599) (19.3051, 61.1431) (19.2564, 61.126) (19.2079, 61.1086) (19.1597, 61.0908) (19.1117, 61.0724) (19.064, 61.0536) (19.0167, 61.0341) (18.9697, 61.014) (18.9231, 60.9935) (18.8766, 60.9725) (18.8304, 60.9513) (18.7843, 60.9298) (18.7385, 60.9079) (18.6931, 60.8852) (18.6485, 60.8613) (18.6137, 60.8409) (18.5881, 60.8246) (18.5713, 60.8134) (18.563, 60.8076) knots -1 -1 -1 -1 -1 -1 -0.98571429 -0.97142857 -0.95714286 -0.94285714 -0.92857143 -0.91428571 -0.9 -0.88571429 -0.87142857 -0.85714286 -0.84285714 -0.82857143 -0.81428571 -0.8 -0.78571429 -0.77142857 -0.75714286 -0.74285714 -0.72857143 -0.71428571 -0.7 -0.68571429 -0.67142857 -0.65714286 -0.64285714 -0.62857143 -0.61428571 -0.6 -0.58571429 -0.57142857 -0.55714286 -0.54285714 -0.52857143 -0.51428571 -0.5 -0.48571429 -0.47142857 -0.45714286 -0.44285714 -0.42857143 -0.41428571 -0.4 -0.38571429 -0.37142857 -0.35714286 -0.34285714 -0.32857143 -0.31428571 -0.3 -0.28571429 -0.27142857 -0.25714286 -0.24285714 -0.22857143 -0.21428571 -0.2 -0.18571429 -0.17142857 -0.15714286 -0.14285714 -0.12857143 -0.11428571 -0.1 -0.08571429 -0.07142857 -0.05714286 -0.04285714 -0.02857143 -0.01428571 0 0 0 0 0 0
  line L29 (18.563, 60.8076) -> (18.5413, 60.7927)
  arc A59 (17.1769, 61.0124) -> (18.5413, 60.7927) centre (17.974, 61.6162) ccw
  arc A60 (17.1769, 61.0124) -> (17.0147, 61.2238) centre (0, 48) ccw
  arc A61 (17.1556, 62.5985) -> (17.0147, 61.2238) centre (17.8043, 61.8374) ccw
  line L30 (17.1556, 62.5985) -> (17.1757, 62.6156)
  spline S30 degree 5 poles (17.1757, 62.6156) (17.1834, 62.6222) (17.1986, 62.6355) (17.2209, 62.656) (17.2497, 62.6843) (17.2843, 62.7212) (17.3179, 62.7592) (17.3509, 62.7977) (17.3836, 62.8367) (17.4161, 62.8759) (17.4484, 62.9153) (17.4803, 62.9551) (17.5119, 62.9953) (17.5429, 63.0359) (17.5735, 63.0771) (17.6036, 63.1187) (17.6333, 63.1607) (17.6627, 63.203) (17.6918, 63.2456) (17.7206, 63.2885) (17.7492, 63.3316) (17.7775, 63.375) (17.8054, 63.4187) (17.8331, 63.4626) (17.8604, 63.5069) (17.8875, 63.5514) (17.9142, 63.5963) (17.9407, 63.6413) (17.9669, 63.6866) (17.9929, 63.7321) (18.0186, 63.7779) (18.044, 63.8239) (18.0692, 63.8701) (18.0941, 63.9165) (18.1188, 63.9632) (18.1432, 64.0101) (18.1673, 64.0572) (18.1912, 64.1045) (18.2149, 64.152) (18.2383, 64.1997) (18.2615, 64.2476) (18.2844, 64.2957) (18.3071, 64.344) (18.3296, 64.3925) (18.3518, 64.4412) (18.3738, 64.49) (18.3956, 64.5391) (18.4171, 64.5883) (18.4384, 64.6377) (18.4595, 64.6873) (18.4804, 64.737) (18.501, 64.787) (18.5214, 64.8371) (18.5416, 64.8873) (18.5615, 64.9377) (18.5813, 64.9883) (18.6008, 65.0391) (18.6201, 65.09) (18.6392, 65.1411) (18.658, 65.1923) (18.6767, 65.2437) (18.6951, 65.2953) (18.7133, 65.3469) (18.7313, 65.3988) (18.7491, 65.4508) (18.7667, 65.5029) (18.784, 65.5552) (18.8012, 65.6076) (18.8181, 65.6602) (18.8348, 65.7129) (18.8514, 65.7658) (18.8644, 65.8081) (18.8741, 65.84) (18.8805, 65.8613) (18.8837, 65.8719) knots 0 0 0 0 0 0 0.01428571 0.02857143 0.04285714 0.05714286 0.07142857 0.08571429 0.1 0.11428571 0.12857143 0.14285714 0.15714286 0.17142857 0.18571429 0.2 0.21428571 0.22857143 0.24285714 0.25714286 0.27142857 0.28571429 0.3 0.31428571 0.32857143 0.34285714 0.35714286 0.37142857 0.38571429 0.4 0.41428571 0.42857143 0.44285714 0.45714286 0.47142857 0.48571429 0.5 0.51428571 0.52857143 0.54285714 0.55714286 0.57142857 0.58571429 0.6 0.61428571 0.62857143 0.64285714 0.65714286 0.67142857 0.68571429 0.7 0.71428571 0.72857143 0.74285714 0.75714286 0.77142857 0.78571429 0.8 0.81428571 0.82857143 0.84285714 0.85714286 0.87142857 0.88571429 0.9 0.91428571 0.92857143 0.94285714 0.95714286 0.97142857 0.98571429 1 1 1 1 1 1
  arc A62 (18.8837, 65.8719) -> (17.8719, 66.8837) centre (0, 48) ccw
  spline S31 degree 5 poles (17.8719, 66.8837) (17.8613, 66.8805) (17.84, 66.8741) (17.8081, 66.8644) (17.7658, 66.8514) (17.7129, 66.8348) (17.6602, 66.8181) (17.6076, 66.8012) (17.5552, 66.784) (17.5029, 66.7667) (17.4508, 66.7491) (17.3988, 66.7313) (17.3469, 66.7133) (17.2953, 66.6951) (17.2437, 66.6767) (17.1923, 66.658) (17.1411, 66.6392) (17.09, 66.6201) (17.0391, 66.6008) (16.9883, 66.5813) (16.9377, 66.5615) (16.8873, 66.5416) (16.8371, 66.5214) (16.787, 66.501) (16.737, 66.4804) (16.6873, 66.4595) (16.6377, 66.4384) (16.5883, 66.4171) (16.5391, 66.3956) (16.49, 66.3738) (16.4412, 66.3518) (16.3925, 66.3296) (16.344, 66.3071) (16.2957, 66.2844) (16.2476, 66.2615) (16.1997, 66.2383) (16.152, 66.2149) (16.1045, 66.1912) (16.0572, 66.1673) (16.0101, 66.1432) (15.9632, 66.1188) (15.9165, 66.0941) (15.8701, 66.0692) (15.8239, 66.044) (15.7779, 66.0186) (15.7321, 65.9929) (15.6866, 65.9669) (15.6413, 65.9407) (15.5963, 65.9142) (15.5514, 65.8875) (15.5069, 65.8604) (15.4626, 65.8331) (15.4187, 65.8054) (15.375, 65.7775) (15.3316, 65.7492) (15.2885, 65.7206) (15.2456, 65.6918) (15.203, 65.6627) (15.1607, 65.6333) (15.1187, 65.6036) (15.0771, 65.5735) (15.0359, 65.5429) (14.9953, 65.5119) (14.9551, 65.4803) (14.9153, 65.4484) (14.8759, 65.4161) (14.8367, 65.3836) (14.7977, 65.3509) (14.7592, 65.3179) (14.7212, 65.2843) (14.6843, 65.2497) (14.656, 65.2209) (14.6355, 65.1986) (14.6222, 65.1834) (14.6156, 65.1757) knots -1 -1 -1 -1 -1 -1 -0.98571429 -0.97142857 -0.95714286 -0.94285714 -0.92857143 -0.91428571 -0.9 -0.88571429 -0.87142857 -0.85714286 -0.84285714 -0.82857143 -0.81428571 -0.8 -0.78571429 -0.77142857 -0.75714286 -0.74285714 -0.72857143 -0.71428571 -0.7 -0.68571429 -0.67142857 -0.65714286 -0.64285714 -0.62857143 -0.61428571 -0.6 -0.58571429 -0.57142857 -0.55714286 -0.54285714 -0.52857143 -0.51428571 -0.5 -0.48571429 -0.47142857 -0.45714286 -0.44285714 -0.42857143 -0.41428571 -0.4 -0.38571429 -0.37142857 -0.35714286 -0.34285714 -0.32857143 -0.31428571 -0.3 -0.28571429 -0.27142857 -0.25714286 -0.24285714 -0.22857143 -0.21428571 -0.2 -0.18571429 -0.17142857 -0.15714286 -0.14285714 -0.12857143 -0.11428571 -0.1 -0.08571429 -0.07142857 -0.05714286 -0.04285714 -0.02857143 -0.01428571 0 0 0 0 0 0
  line L31 (14.6156, 65.1757) -> (14.5985, 65.1556)
  arc A63 (13.2238, 65.0147) -> (14.5985, 65.1556) centre (13.8374, 65.8043) ccw
  arc A64 (13.2238, 65.0147) -> (13.0124, 65.1769) centre (0, 48) ccw
  arc A65 (12.7927, 66.5413) -> (13.0124, 65.1769) centre (13.6162, 65.974) ccw
  line L32 (12.7927, 66.5413) -> (12.8076, 66.563)
  spline S32 degree 5 poles (12.8076, 66.563) (12.8134, 66.5713) (12.8246, 66.5881) (12.8409, 66.6137) (12.8613, 66.6485) (12.8852, 66.6931) (12.9079, 66.7385) (12.9298, 66.7843) (12.9513, 66.8304) (12.9725, 66.8766) (12.9935, 66.9231) (13.014, 66.9697) (13.0341, 67.0167) (13.0536, 67.064) (13.0724, 67.1117) (13.0908, 67.1597) (13.1086, 67.2079) (13.126, 67.2564) (13.1431, 67.3051) (13.1599, 67.354) (13.1763, 67.403) (13.1924, 67.4522) (13.2081, 67.5017) (13.2234, 67.5513) (13.2384, 67.6011) (13.253, 67.6512) (13.2672, 67.7014) (13.2811, 67.7517) (13.2947, 67.8023) (13.308, 67.853) (13.321, 67.9038) (13.3337, 67.9548) (13.346, 68.006) (13.3581, 68.0573) (13.3698, 68.1087) (13.3812, 68.1603) (13.3924, 68.2121) (13.4032, 68.264) (13.4138, 68.316) (13.4241, 68.3681) (13.4341, 68.4204) (13.4438, 68.4728) (13.4532, 68.5253) (13.4623, 68.578) (13.4712, 68.6307) (13.4798, 68.6836) (13.4882, 68.7366) (13.4962, 68.7898) (13.504, 68.843) (13.5115, 68.8963) (13.5188, 68.9498) (13.5258, 69.0034) (13.5325, 69.057) (13.539, 69.1108) (13.5453, 69.1647) (13.5512, 69.2187) (13.5569, 69.2727) (13.5624, 69.3269) (13.5676, 69.3812) (13.5726, 69.4356) (13.5773, 69.49) (13.5817, 69.5446) (13.586, 69.5992) (13.5899, 69.654) (13.5936, 69.7088) (13.5971, 69.7637) (13.6004, 69.8187) (13.6034, 69.8738) (13.6061, 69.9289) (13.6086, 69.9842) (13.6109, 70.0395) (13.6125, 70.0838) (13.6137, 70.1171) (13.6143, 70.1393) (13.6147, 70.1504) knots 0 0 0 0 0 0 0.01428571 0.02857143 0.04285714 0.05714286 0.07142857 0.08571429 0.1 0.11428571 0.12857143 0.14285714 0.15714286 0.17142857 0.18571429 0.2 0.21428571 0.22857143 0.24285714 0.25714286 0.27142857 0.28571429 0.3 0.31428571 0.32857143 0.34285714 0.35714286 0.37142857 0.38571429 0.4 0.41428571 0.42857143 0.44285714 0.45714286 0.47142857 0.48571429 0.5 0.51428571 0.52857143 0.54285714 0.55714286 0.57142857 0.58571429 0.6 0.61428571 0.62857143 0.64285714 0.65714286 0.67142857 0.68571429 0.7 0.71428571 0.72857143 0.74285714 0.75714286 0.77142857 0.78571429 0.8 0.81428571 0.82857143 0.84285714 0.85714286 0.87142857 0.88571429 0.9 0.91428571 0.92857143 0.94285714 0.95714286 0.97142857 0.98571429 1 1 1 1 1 1
  arc A66 (13.6147, 70.1504) -> (12.3755, 70.8659) centre (0, 48) ccw
  spline S33 degree 5 poles (12.3755, 70.8659) (12.366, 70.86) (12.3471, 70.8483) (12.3189, 70.8307) (12.2813, 70.8071) (12.2345, 70.7775) (12.188, 70.7477) (12.1416, 70.7177) (12.0954, 70.6876) (12.0493, 70.6573) (12.0035, 70.6268) (11.9579, 70.5962) (11.9125, 70.5654) (11.8673, 70.5344) (11.8223, 70.5033) (11.7775, 70.472) (11.7329, 70.4405) (11.6885, 70.4088) (11.6443, 70.377) (11.6003, 70.345) (11.5565, 70.3129) (11.513, 70.2805) (11.4697, 70.248) (11.4265, 70.2154) (11.3837, 70.1825) (11.341, 70.1495) (11.2986, 70.1163) (11.2564, 70.0829) (11.2144, 70.0494) (11.1726, 70.0157) (11.1311, 69.9818) (11.0899, 69.9477) (11.0488, 69.9135) (11.0081, 69.879) (10.9675, 69.8444) (10.9273, 69.8096) (10.8873, 69.7747) (10.8475, 69.7395) (10.808, 69.7042) (10.7687, 69.6687) (10.7298, 69.633) (10.6911, 69.5971) (10.6527, 69.561) (10.6146, 69.5247) (10.5767, 69.4882) (10.5392, 69.4516) (10.5019, 69.4147) (10.4649, 69.3777) (10.4283, 69.3404) (10.3919, 69.303) (10.3559, 69.2653) (10.3202, 69.2275) (10.2849, 69.1894) (10.2499, 69.1511) (10.2153, 69.1125) (10.1811, 69.0738) (10.1471, 69.0348) (10.1135, 68.9957) (10.0803, 68.9563) (10.0474, 68.9168) (10.015, 68.8769) (9.9832, 68.8367) (9.9519, 68.7962) (9.9213, 68.7554) (9.8911, 68.7142) (9.8614, 68.6728) (9.8319, 68.6313) (9.8028, 68.5897) (9.7741, 68.5478) (9.7461, 68.5055) (9.7194, 68.4625) (9.6995, 68.4274) (9.6855, 68.4005) (9.6765, 68.3824) (9.6722, 68.3732) knots -1 -1 -1 -1 -1 -1 -0.98571429 -0.97142857 -0.95714286 -0.94285714 -0.92857143 -0.91428571 -0.9 -0.88571429 -0.87142857 -0.85714286 -0.84285714 -0.82857143 -0.81428571 -0.8 -0.78571429 -0.77142857 -0.75714286 -0.74285714 -0.72857143 -0.71428571 -0.7 -0.68571429 -0.67142857 -0.65714286 -0.64285714 -0.62857143 -0.61428571 -0.6 -0.58571429 -0.57142857 -0.55714286 -0.54285714 -0.52857143 -0.51428571 -0.5 -0.48571429 -0.47142857 -0.45714286 -0.44285714 -0.42857143 -0.41428571 -0.4 -0.38571429 -0.37142857 -0.35714286 -0.34285714 -0.32857143 -0.31428571 -0.3 -0.28571429 -0.27142857 -0.25714286 -0.24285714 -0.22857143 -0.21428571 -0.2 -0.18571429 -0.17142857 -0.15714286 -0.14285714 -0.12857143 -0.11428571 -0.1 -0.08571429 -0.07142857 -0.05714286 -0.04285714 -0.02857143 -0.01428571 0 0 0 0 0 0
  line L33 (9.6722, 68.3732) -> (9.6609, 68.3494)
  arc A67 (8.3695, 67.8575) -> (9.6609, 68.3494) centre (8.7578, 68.779) ccw
  arc A68 (8.3695, 67.8575) -> (8.1233, 67.9595) centre (0, 48) ccw
  arc A69 (7.5579, 69.2205) -> (8.1233, 67.9595) centre (8.5002, 68.8857) ccw
  line L34 (7.5579, 69.2205) -> (7.5668, 69.2453)
  spline S34 degree 5 poles (7.5668, 69.2453) (7.5702, 69.2549) (7.5767, 69.274) (7.5858, 69.3029) (7.5965, 69.3419) (7.608, 69.3911) (7.6182, 69.4408) (7.6275, 69.4907) (7.6363, 69.5408) (7.6449, 69.591) (7.6531, 69.6412) (7.6609, 69.6916) (7.6681, 69.7422) (7.6746, 69.7929) (7.6805, 69.8439) (7.6858, 69.895) (7.6906, 69.9462) (7.6948, 69.9975) (7.6988, 70.049) (7.7023, 70.1005) (7.7055, 70.1521) (7.7083, 70.2039) (7.7106, 70.2557) (7.7126, 70.3076) (7.7141, 70.3596) (7.7153, 70.4117) (7.7161, 70.4639) (7.7165, 70.5161) (7.7165, 70.5685) (7.7162, 70.6209) (7.7156, 70.6733) (7.7146, 70.7259) (7.7133, 70.7785) (7.7117, 70.8312) (7.7097, 70.8839) (7.7074, 70.9367) (7.7048, 70.9896) (7.7018, 71.0425) (7.6986, 71.0955) (7.695, 71.1485) (7.6911, 71.2016) (7.6869, 71.2547) (7.6824, 71.3079) (7.6777, 71.3611) (7.6726, 71.4144) (7.6672, 71.4677) (7.6615, 71.521) (7.6556, 71.5744) (7.6493, 71.6279) (7.6428, 71.6814) (7.636, 71.7349) (7.6289, 71.7884) (7.6215, 71.842) (7.6138, 71.8956) (7.6059, 71.9493) (7.5977, 72.003) (7.5892, 72.0567) (7.5805, 72.1104) (7.5714, 72.1642) (7.5622, 72.218) (7.5526, 72.2718) (7.5428, 72.3257) (7.5327, 72.3796) (7.5224, 72.4335) (7.5118, 72.4874) (7.501, 72.5413) (7.4899, 72.5953) (7.4785, 72.6492) (7.4669, 72.7032) (7.455, 72.7573) (7.4429, 72.8113) (7.433, 72.8545) (7.4255, 72.8869) (7.4204, 72.9086) (7.4178, 72.9194) knots 0 0 0 0 0 0 0.01428571 0.02857143 0.04285714 0.05714286 0.07142857 0.08571429 0.1 0.11428571 0.12857143 0.14285714 0.15714286 0.17142857 0.18571429 0.2 0.21428571 0.22857143 0.24285714 0.25714286 0.27142857 0.28571429 0.3 0.31428571 0.32857143 0.34285714 0.35714286 0.37142857 0.38571429 0.4 0.41428571 0.42857143 0.44285714 0.45714286 0.47142857 0.48571429 0.5 0.51428571 0.52857143 0.54285714 0.55714286 0.57142857 0.58571429 0.6 0.61428571 0.62857143 0.64285714 0.65714286 0.67142857 0.68571429 0.7 0.71428571 0.72857143 0.74285714 0.75714286 0.77142857 0.78571429 0.8 0.81428571 0.82857143 0.84285714 0.85714286 0.87142857 0.88571429 0.9 0.91428571 0.92857143 0.94285714 0.95714286 0.97142857 0.98571429 1 1 1 1 1 1
  arc A70 (7.4178, 72.9194) -> (6.0357, 73.2897) centre (0, 48) ccw
  spline S35 degree 5 poles (6.0357, 73.2897) (6.0281, 73.2816) (6.0128, 73.2655) (5.9901, 73.2411) (5.9599, 73.2086) (5.9224, 73.1679) (5.8851, 73.1271) (5.8481, 73.0861) (5.8112, 73.0451) (5.7746, 73.0039) (5.7383, 72.9626) (5.7021, 72.9212) (5.6662, 72.8797) (5.6306, 72.8381) (5.5952, 72.7963) (5.56, 72.7545) (5.525, 72.7125) (5.4903, 72.6705) (5.4559, 72.6283) (5.4217, 72.586) (5.3878, 72.5436) (5.3541, 72.5011) (5.3206, 72.4585) (5.2874, 72.4158) (5.2545, 72.373) (5.2218, 72.33) (5.1895, 72.287) (5.1573, 72.2438) (5.1255, 72.2006) (5.0939, 72.1572) (5.0625, 72.1137) (5.0315, 72.0701) (5.0007, 72.0264) (4.9703, 71.9826) (4.9401, 71.9387) (4.9102, 71.8947) (4.8806, 71.8505) (4.8513, 71.8063) (4.8223, 71.7619) (4.7935, 71.7175) (4.7651, 71.6729) (4.7371, 71.6282) (4.7093, 71.5834) (4.6819, 71.5385) (4.6548, 71.4935) (4.628, 71.4484) (4.6015, 71.4031) (4.5754, 71.3578) (4.5496, 71.3123) (4.5242, 71.2667) (4.4992, 71.221) (4.4745, 71.1752) (4.4502, 71.1293) (4.4264, 71.0832) (4.4029, 71.037) (4.3799, 70.9908) (4.3572, 70.9444) (4.3348, 70.8979) (4.3129, 70.8512) (4.2914, 70.8045) (4.2704, 70.7576) (4.25, 70.7106) (4.2304, 70.6633) (4.2113, 70.6159) (4.1929, 70.5684) (4.1748, 70.5207) (4.1571, 70.473) (4.1398, 70.4252) (4.1229, 70.3773) (4.1068, 70.3292) (4.0922, 70.2808) (4.082, 70.2417) (4.0754, 70.2122) (4.0715, 70.1923) (4.0696, 70.1824) knots -1 -1 -1 -1 -1 -1 -0.98571429 -0.97142857 -0.95714286 -0.94285714 -0.92857143 -0.91428571 -0.9 -0.88571429 -0.87142857 -0.85714286 -0.84285714 -0.82857143 -0.81428571 -0.8 -0.78571429 -0.77142857 -0.75714286 -0.74285714 -0.72857143 -0.71428571 -0.7 -0.68571429 -0.67142857 -0.65714286 -0.64285714 -0.62857143 -0.61428571 -0.6 -0.58571429 -0.57142857 -0.55714286 -0.54285714 -0.52857143 -0.51428571 -0.5 -0.48571429 -0.47142857 -0.45714286 -0.44285714 -0.42857143 -0.41428571 -0.4 -0.38571429 -0.37142857 -0.35714286 -0.34285714 -0.32857143 -0.31428571 -0.3 -0.28571429 -0.27142857 -0.25714286 -0.24285714 -0.22857143 -0.21428571 -0.2 -0.18571429 -0.17142857 -0.15714286 -0.14285714 -0.12857143 -0.11428571 -0.1 -0.08571429 -0.07142857 -0.05714286 -0.04285714 -0.02857143 -0.01428571 0 0 0 0 0 0
  line L35 (4.0696, 70.1824) -> (4.0649, 70.1564)
  arc A71 (2.9448, 69.347) -> (4.0649, 70.1564) centre (3.0814, 70.3377) ccw
  arc A72 (2.9448, 69.347) -> (2.6806, 69.3818) centre (0, 48) ccw
  arc A73 (1.8082, 70.4535) -> (2.6806, 69.3818) centre (2.805, 70.3741) ccw
  line L36 (1.8082, 70.4535) -> (1.8102, 70.4799)
  spline S36 degree 5 poles (1.8102, 70.4799) (1.8111, 70.4899) (1.8124, 70.5101) (1.8137, 70.5404) (1.814, 70.5808) (1.8123, 70.6313) (1.8093, 70.6819) (1.8054, 70.7326) (1.801, 70.7832) (1.7962, 70.8339) (1.7911, 70.8846) (1.7856, 70.9353) (1.7795, 70.986) (1.7727, 71.0367) (1.7652, 71.0874) (1.7571, 71.1381) (1.7484, 71.1889) (1.7393, 71.2396) (1.7297, 71.2903) (1.7198, 71.341) (1.7095, 71.3916) (1.6988, 71.4423) (1.6877, 71.493) (1.6762, 71.5436) (1.6642, 71.5943) (1.6518, 71.6449) (1.6391, 71.6955) (1.6259, 71.7461) (1.6124, 71.7966) (1.5986, 71.8472) (1.5844, 71.8977) (1.5699, 71.9482) (1.555, 71.9987) (1.5398, 72.0491) (1.5242, 72.0996) (1.5083, 72.15) (1.4921, 72.2004) (1.4756, 72.2507) (1.4587, 72.301) (1.4415, 72.3513) (1.424, 72.4016) (1.4062, 72.4518) (1.3881, 72.502) (1.3697, 72.5522) (1.351, 72.6024) (1.3321, 72.6525) (1.3128, 72.7025) (1.2932, 72.7526) (1.2733, 72.8026) (1.2532, 72.8525) (1.2327, 72.9025) (1.212, 72.9523) (1.191, 73.0022) (1.1697, 73.052) (1.1482, 73.1018) (1.1264, 73.1515) (1.1043, 73.2012) (1.0819, 73.2509) (1.0593, 73.3005) (1.0364, 73.35) (1.0133, 73.3995) (0.9898, 73.449) (0.9662, 73.4985) (0.9422, 73.5478) (0.9181, 73.5972) (0.8936, 73.6465) (0.8689, 73.6957) (0.844, 73.7449) (0.8188, 73.7941) (0.7933, 73.8432) (0.7676, 73.8922) (0.7469, 73.9314) (0.7312, 73.9608) (0.7207, 73.9804) (0.7155, 73.9902) knots 0 0 0 0 0 0 0.01428571 0.02857143 0.04285714 0.05714286 0.07142857 0.08571429 0.1 0.11428571 0.12857143 0.14285714 0.15714286 0.17142857 0.18571429 0.2 0.21428571 0.22857143 0.24285714 0.25714286 0.27142857 0.28571429 0.3 0.31428571 0.32857143 0.34285714 0.35714286 0.37142857 0.38571429 0.4 0.41428571 0.42857143 0.44285714 0.45714286 0.47142857 0.48571429 0.5 0.51428571 0.52857143 0.54285714 0.55714286 0.57142857 0.58571429 0.6 0.61428571 0.62857143 0.64285714 0.65714286 0.67142857 0.68571429 0.7 0.71428571 0.72857143 0.74285714 0.75714286 0.77142857 0.78571429 0.8 0.81428571 0.82857143 0.84285714 0.85714286 0.87142857 0.88571429 0.9 0.91428571 0.92857143 0.94285714 0.95714286 0.97142857 0.98571429 1 1 1 1 1 1
  arc A74 (0.7155, 73.9902) -> (-0.7155, 73.9902) centre (0, 48) ccw